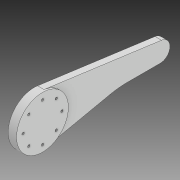
# Autodesk Inventor part: TestArm
Saved by Autodesk Inventor 2020 (Build 240168000, 168)
## iProperties
Created: 2021-04-06
Part Number: TestArm
Material: Generic
Document SubType Name: Modeling
Designer: DDeGo
Density: 1 g/cm^3
Appearance: Default
Author: DDeGo
Autodesk Inventor part; units mm, degrees
ref_plane "YZ Plane" through (0, 0, 0) normal (1, 0, 0) x (0, 1, 0)
ref_plane "XZ Plane" through (0, 0, 0) normal (0, 1, 0) x (-1, 0, 0)
ref_plane "XY Plane" through (0, 0, 0) normal (0, 0, 1) x (1, 0, 0)
sketch "Sketch1" plane through (0, 0, 0) normal (1, 0, 0) x (0, 1, 0)
  circle A0 centre (0, 0) radius 30 construction
  arc A1 (39.6331, -5.4054) -> (-39.1177, -8.3551) centre (0, 0) ccw
  arc A2 (-15, -185) -> (14.8624, -187.027) centre (0, -185) ccw
  line L0 (39.6331, -5.4054) -> (14.8624, -187.027)
  line L1 (0, 0) -> (0, -185) construction
  line L2 (74.7174, 40) -> (-69.809, 40) construction
  line L3 (-69.809, 40) -> (-69.809, -200) construction
  line L4 (-69.809, -200) -> (74.7174, -200) construction
  line L5 (74.7174, -200) -> (74.7174, 40) construction
  line L6 (-15, -185) -> (-15, -135)
  line L7 (-17.8676, -107.846) -> (-39.1177, -8.3551)
  arc A3 (-15, -135) -> (-17.8676, -107.846) centre (-145, -135) ccw
  circle A4 centre (0, -30) radius 1.75
  circle A5 centre (21.2132, -21.2132) radius 1.75
  circle A6 centre (30, 0) radius 1.75
  circle A7 centre (21.2132, 21.2132) radius 1.75
  circle A8 centre (0, 30) radius 1.75
  circle A9 centre (-21.2132, 21.2132) radius 1.75
  circle A10 centre (-30, 0) radius 1.75
  circle A11 centre (-21.2132, -21.2132) radius 1.75
  dimension "d0" = 60
  dimension "d1" = 80
  dimension "d2" = 30
  dimension "d3" = 240
  dimension "d4" = 130
  dimension "d5" = 50
  dimension "d6" = 3.5
  dimension "d9" = 360
  dimension "d15" = 185
  constraints: 16 end point, 11 centre point, 8 tangent, 6 point on circle, 2 coincident, 2 parallel, 2 vertical, 1 horizontal, 1 perpendicular, 1 point on line, 1 vertical alignment, 19 other
  measures "d1" diameter of A1
  measures "d2" diameter of A2
  measures "d3" distance between parallel lines of L2 L4
  measures "d4" radius of A3
  measures "d5" distance of L6.start L6.end
  measures "d6" diameter of A4
  measures "d15" distance of L1.start L1.end
extrude "Extrusion1" add sketch "Sketch1" along normal blind 10
sketch "Sketch2" plane through (10, 0, 0) normal (1, 0, 0) x (0, 0, -1)
  arc A0 (135, -15) -> (107.846, -17.8676) centre (135, -145) ccw projected
  line L0 (135, -15) -> (185, -15) projected
  arc A1 (185, -15) -> (187.027, 14.8624) centre (185, 0) ccw projected
  line L1 (187.027, 14.8624) -> (5.4054, 39.6331) projected
  arc A2 (5.4054, 39.6331) -> (8.3551, -39.1177) centre (0, 0) ccw projected
  line L2 (8.3551, -39.1177) -> (107.846, -17.8676) projected
  circle A3 centre (30, 0) radius 1.75 projected
  circle A4 centre (21.2132, -21.2132) radius 1.75 projected
  circle A5 centre (0, -30) radius 1.75 projected
  circle A6 centre (-21.2132, -21.2132) radius 1.75 projected
  circle A7 centre (-30, 0) radius 1.75 projected
  circle A8 centre (-21.2132, 21.2132) radius 1.75 projected
  circle A9 centre (0, 30) radius 1.75 projected
  circle A10 centre (21.2132, 21.2132) radius 1.75 projected
  arc A11 (5.4054, 39.6331) -> (8.3551, -39.1177) centre (0, 0) ccw projected
  circle A12 centre (0, 0) radius 40
  point P0 (5.4054, 39.6331)
  constraints: 1 coincident, 3 other
extrude "Extrusion2" add sketch "Sketch2" along normal blind 3 contours A2 A12
body "Solid1"
